Autodesk Inventor part; units mm, degrees
(part 2 of 2)
  spline S259 degree 2 poles (-5.2071, -17.5156) (-5.4392, -17.6614) (-5.9159, -17.7602) (-6.2865, -17.7602) knots 0 0 0 1 2 2 2
  line L295 (-6.2865, -17.7602) -> (-6.9879, -17.7602)
  line L296 (-6.9879, -17.7602) -> (-6.9879, -14.7122)
  line L297 (-6.9879, -14.7122) -> (-6.2939, -14.7122)
  spline S260 degree 2 poles (-6.2939, -14.7122) (-5.8641, -14.7122) (-5.375, -14.8406) (-5.2021, -14.9542) knots 0 0 0 1 2 2 2
  spline S261 degree 2 poles (-5.2021, -14.9542) (-4.9082, -15.1494) (-4.5846, -15.794) (-4.5846, -16.2386) knots 0 0 0 1 2 2 2
  spline S262 degree 2 poles (-5.007, -16.2337) (-5.007, -15.8829) (-5.2392, -15.3865) (-5.4689, -15.2457) knots 0 0 0 1 2 2 2
  spline S263 degree 2 poles (-5.4689, -15.2457) (-5.6319, -15.1494) (-5.9999, -15.0629) (-6.2741, -15.0629) knots 0 0 0 1 2 2 2
  line L298 (-6.2741, -15.0629) -> (-6.5829, -15.0629)
  line L299 (-6.5829, -15.0629) -> (-6.5829, -17.4094)
  line L300 (-6.5829, -17.4094) -> (-6.2741, -17.4094)
  spline S264 degree 2 poles (-6.2741, -17.4094) (-6.0049, -17.4094) (-5.5973, -17.323) (-5.4318, -17.2069) knots 0 0 0 1 2 2 2
  spline S265 degree 2 poles (-5.4318, -17.2069) (-5.2194, -17.0636) (-5.007, -16.5894) (-5.007, -16.2337) knots 0 0 0 1 2 2 2
  line L301 (-3.115, -16.6116) -> (-4.2684, -16.6116)
  line L302 (-4.2684, -16.6116) -> (-4.2684, -16.2411)
  line L303 (-4.2684, -16.2411) -> (-3.115, -16.2411)
  line L304 (-3.115, -16.2411) -> (-3.115, -16.6116)
  line L305 (-0.9833, -17.7602) -> (-2.4703, -17.7602)
  line L306 (-2.4703, -17.7602) -> (-2.4703, -17.4489)
  line L307 (-2.4703, -17.4489) -> (-1.917, -17.4489)
  line L308 (-1.917, -17.4489) -> (-1.917, -15.4062)
  line L309 (-1.917, -15.4062) -> (-2.4703, -15.4062)
  line L310 (-2.4703, -15.4062) -> (-2.4703, -15.1271)
  spline S266 degree 2 poles (-2.4703, -15.1271) (-2.1566, -15.1271) (-1.8602, -14.9493) (-1.8404, -14.7023) knots 0 0 0 1 2 2 2
  line L311 (-1.8404, -14.7023) -> (-1.5243, -14.7023)
  line L312 (-1.5243, -14.7023) -> (-1.5243, -17.4489)
  line L313 (-1.5243, -17.4489) -> (-0.9833, -17.4489)
  line L314 (-0.9833, -17.4489) -> (-0.9833, -17.7602)
  line L315 (1.457, -17.7602) -> (-0.4226, -17.7602)
  line L316 (-0.4226, -17.7602) -> (-0.4226, -17.3279)
  spline S267 degree 2 poles (-0.4226, -17.3279) (-0.2201, -17.1377) (0.1405, -16.7845) (0.3134, -16.5943) knots 0 0 0 1 2 2 2
  spline S268 degree 2 poles (0.3134, -16.5943) (0.6617, -16.2115) (0.9161, -15.752) (0.9161, -15.5075) knots 0 0 0 1 2 2 2
  spline S269 degree 2 poles (0.9161, -15.5075) (0.9161, -15.3791) (0.8371, -15.1864) (0.7654, -15.1247) knots 0 0 0 1 2 2 2
  spline S270 degree 2 poles (0.7654, -15.1247) (0.6938, -15.0629) (0.5061, -15.0012) (0.3925, -15.0012) knots 0 0 0 1 2 2 2
  spline S271 degree 2 poles (0.3925, -15.0012) (0.2838, -15.0012) (0.0615, -15.0555) (-0.0398, -15.0975) knots 0 0 0 1 2 2 2
  spline S272 degree 2 poles (-0.0398, -15.0975) (-0.1262, -15.1321) (-0.2868, -15.2309) (-0.3362, -15.2654) knots 0 0 0 1 2 2 2
  line L317 (-0.3362, -15.2654) -> (-0.3584, -15.2654)
  line L318 (-0.3584, -15.2654) -> (-0.3584, -14.8307)
  spline S273 degree 2 poles (-0.3584, -14.8307) (-0.2324, -14.769) (0.2196, -14.6479) (0.4221, -14.6479) knots 0 0 0 1 2 2 2
  spline S274 degree 2 poles (0.4221, -14.6479) (0.8494, -14.6479) (1.3311, -15.1) (1.3311, -15.4853) knots 0 0 0 1 2 2 2
  spline S275 degree 2 poles (1.3311, -15.4853) (1.3311, -15.6656) (1.2471, -15.9669) (1.173, -16.0954) knots 0 0 0 1 2 2 2
  spline S276 degree 2 poles (1.173, -16.0954) (1.0989, -16.2288) (0.884, -16.4906) (0.7654, -16.6165) knots 0 0 0 1 2 2 2
  spline S277 degree 2 poles (0.7654, -16.6165) (0.5728, -16.8265) (0.101, -17.276) (-0.0398, -17.4069) knots 0 0 0 1 2 2 2
  line L319 (-0.0398, -17.4069) -> (1.457, -17.4069)
  line L320 (1.457, -17.4069) -> (1.457, -17.7602)
  line L321 (3.7443, -17.7602) -> (1.8646, -17.7602)
  line L322 (1.8646, -17.7602) -> (1.8646, -17.3279)
  spline S278 degree 2 poles (1.8646, -17.3279) (2.0671, -17.1377) (2.4278, -16.7845) (2.6007, -16.5943) knots 0 0 0 1 2 2 2
  spline S279 degree 2 poles (2.6007, -16.5943) (2.9489, -16.2115) (3.2034, -15.752) (3.2034, -15.5075) knots 0 0 0 1 2 2 2
  spline S280 degree 2 poles (3.2034, -15.5075) (3.2034, -15.3791) (3.1243, -15.1864) (3.0527, -15.1247) knots 0 0 0 1 2 2 2
  spline S281 degree 2 poles (3.0527, -15.1247) (2.981, -15.0629) (2.7933, -15.0012) (2.6797, -15.0012) knots 0 0 0 1 2 2 2
  spline S282 degree 2 poles (2.6797, -15.0012) (2.571, -15.0012) (2.3487, -15.0555) (2.2475, -15.0975) knots 0 0 0 1 2 2 2
  spline S283 degree 2 poles (2.2475, -15.0975) (2.161, -15.1321) (2.0005, -15.2309) (1.9511, -15.2654) knots 0 0 0 1 2 2 2
  line L323 (1.9511, -15.2654) -> (1.9288, -15.2654)
  line L324 (1.9288, -15.2654) -> (1.9288, -14.8307)
  spline S284 degree 2 poles (1.9288, -14.8307) (2.0548, -14.769) (2.5068, -14.6479) (2.7093, -14.6479) knots 0 0 0 1 2 2 2
  spline S285 degree 2 poles (2.7093, -14.6479) (3.1367, -14.6479) (3.6183, -15.1) (3.6183, -15.4853) knots 0 0 0 1 2 2 2
  spline S286 degree 2 poles (3.6183, -15.4853) (3.6183, -15.6656) (3.5343, -15.9669) (3.4602, -16.0954) knots 0 0 0 1 2 2 2
  spline S287 degree 2 poles (3.4602, -16.0954) (3.3861, -16.2288) (3.1712, -16.4906) (3.0527, -16.6165) knots 0 0 0 1 2 2 2
  spline S288 degree 2 poles (3.0527, -16.6165) (2.86, -16.8265) (2.3882, -17.276) (2.2475, -17.4069) knots 0 0 0 1 2 2 2
  line L325 (2.2475, -17.4069) -> (3.7443, -17.4069)
  line L326 (3.7443, -17.4069) -> (3.7443, -17.7602)
  point P0 (0, 0)
  constraints: 4 other
extrude "Extrusion2" cut sketch "Sketch2" against normal blind 1
body "Solid1"
